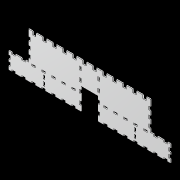
# Autodesk Inventor part: AluminumTopPlate
Saved by Autodesk Inventor 2021 (Build 250183000, 183)
## iProperties
Created: 2021-03-05
Part Number: AluminumTopPlate
Material: Aluminum 6061
Document SubType Name: Modeling
Designer: M3rob
Density: 2.7 g/cm^3
Appearance: Aluminum - Flat
Mass: 6715.1 g
Surface Area: 6765.43 cm^2
Volume: 2487.07 cm^3
Author: M3rob
Autodesk Inventor part; units mm, degrees
ref_plane "YZ Plane" through (0, 0, 0) normal (1, 0, 0) x (0, 1, 0)
ref_plane "XZ Plane" through (0, 0, 0) normal (0, 1, 0) x (-1, 0, 0)
ref_plane "XY Plane" through (0, 0, 0) normal (0, 0, 1) x (1, 0, 0)
sketch "Sketch1" plane through (0, 0, 0) normal (0, 0, 1) x (1, 0, 0)
  line L0 (-527.05, -334.01) -> (-527.05, 34.29) projected
  line L1 (-654.05, 34.29) -> (-654.05, -334.01) projected
  line L2 (-1206.5, -6.35) -> (-654.05, -6.35)
  line L3 (-1206.5, -6.35) -> (-1206.5, 120.65)
  line L4 (-1206.5, 120.65) -> (-1054.1, 120.65)
  line L5 (-1054.1, 120.65) -> (-1054.1, 339.09)
  line L6 (-1054.1, 339.09) -> (-127, 339.09)
  line L7 (-127, 339.09) -> (-127, 120.65)
  line L8 (-127, 120.65) -> (25.4, 120.65)
  line L9 (25.4, 120.65) -> (25.4, -6.35)
  line L10 (25.4, -6.35) -> (-527.05, -6.35)
  line L11 (-654.05, -6.35) -> (-654.05, 161.29)
  line L12 (-654.05, 161.29) -> (-527.05, 161.29)
  line L13 (-527.05, 161.29) -> (-527.05, -6.35)
  line L14 (-946.15, 339.09) -> (-920.75, 339.09) projected
  line L15 (-946.15, 339.09) -> (-946.15, 313.69) projected
  line L16 (-920.75, 313.69) -> (-946.15, 313.69) projected
  line L17 (-920.75, 339.09) -> (-920.75, 313.69) projected
  line L18 (-920.75, 339.09) -> (-869.95, 339.09) projected
  line L19 (-920.75, 339.09) -> (-920.75, 313.69) projected
  line L20 (-869.95, 313.69) -> (-920.75, 313.69) projected
  line L21 (-869.95, 339.09) -> (-869.95, 313.69) projected
  line L22 (-869.95, 339.09) -> (-844.55, 339.09) projected
  line L23 (-869.95, 339.09) -> (-869.95, 313.69) projected
  line L24 (-844.55, 313.69) -> (-869.95, 313.69) projected
  line L25 (-844.55, 339.09) -> (-844.55, 313.69) projected
  line L26 (-828.675, 339.09) -> (-828.675, 313.69) projected
  line L27 (-844.55, 339.09) -> (-825.8937, 339.09) projected
  line L28 (-844.55, 339.09) -> (-844.55, 313.69) projected
  line L29 (-825.8937, 313.69) -> (-844.55, 313.69) projected
  line L30 (-825.8937, 339.09) -> (-825.8937, 313.69) projected
  line L31 (-812.4063, 339.09) -> (-812.4063, 313.69) projected
  line L32 (-825.8937, 339.09) -> (-812.4063, 339.09) projected
  line L33 (-825.8937, 339.09) -> (-825.8937, 313.69) projected
  line L34 (-812.4063, 313.69) -> (-825.8937, 313.69) projected
  line L35 (-812.4063, 339.09) -> (-812.4063, 313.69) projected
  line L36 (-793.75, 339.09) -> (-793.75, 313.69) projected
  line L37 (-812.4063, 339.09) -> (-793.75, 339.09) projected
  line L38 (-812.4063, 339.09) -> (-812.4063, 313.69) projected
  line L39 (-793.75, 313.69) -> (-812.4063, 313.69) projected
  line L40 (-793.75, 339.09) -> (-793.75, 313.69) projected
  line L41 (-793.75, 339.09) -> (-768.35, 339.09) projected
  line L42 (-793.75, 339.09) -> (-793.75, 313.69) projected
  line L43 (-768.35, 313.69) -> (-793.75, 313.69) projected
  line L44 (-768.35, 339.09) -> (-768.35, 313.69) projected
  line L45 (-768.35, 339.09) -> (-717.55, 339.09) projected
  line L46 (-768.35, 339.09) -> (-768.35, 313.69) projected
  line L47 (-717.55, 313.69) -> (-768.35, 313.69) projected
  line L48 (-717.55, 339.09) -> (-717.55, 313.69) projected
  line L49 (-717.55, 339.09) -> (-692.15, 339.09) projected
  line L50 (-717.55, 339.09) -> (-717.55, 313.69) projected
  line L51 (-692.15, 313.69) -> (-717.55, 313.69) projected
  line L52 (-692.15, 339.09) -> (-692.15, 313.69) projected
  line L53 (-692.15, 339.09) -> (-641.35, 339.09) projected
  line L54 (-692.15, 339.09) -> (-692.15, 313.69) projected
  line L55 (-641.35, 313.69) -> (-692.15, 313.69) projected
  line L56 (-641.35, 339.09) -> (-641.35, 313.69) projected
  line L57 (-641.35, 339.09) -> (-615.95, 339.09) projected
  line L58 (-641.35, 339.09) -> (-641.35, 313.69) projected
  line L59 (-615.95, 313.69) -> (-641.35, 313.69) projected
  line L60 (-615.95, 339.09) -> (-615.95, 313.69) projected
  line L61 (-600.075, 339.09) -> (-600.075, 313.69) projected
  line L62 (-615.95, 339.09) -> (-597.2937, 339.09) projected
  line L63 (-615.95, 339.09) -> (-615.95, 313.69) projected
  line L64 (-597.2937, 313.69) -> (-615.95, 313.69) projected
  line L65 (-597.2937, 339.09) -> (-597.2937, 313.69) projected
  line L66 (-565.15, 339.09) -> (-539.75, 339.09) projected
  line L67 (-565.15, 339.09) -> (-565.15, 313.69) projected
  line L68 (-539.75, 313.69) -> (-565.15, 313.69) projected
  line L69 (-539.75, 339.09) -> (-539.75, 313.69) projected
  line L70 (-488.95, 339.09) -> (-463.55, 339.09) projected
  line L71 (-488.95, 339.09) -> (-488.95, 313.69) projected
  line L72 (-463.55, 313.69) -> (-488.95, 313.69) projected
  line L73 (-463.55, 339.09) -> (-463.55, 313.69) projected
  line L74 (-412.75, 339.09) -> (-387.35, 339.09) projected
  line L75 (-412.75, 339.09) -> (-412.75, 313.69) projected
  line L76 (-387.35, 313.69) -> (-412.75, 313.69) projected
  line L77 (-387.35, 339.09) -> (-387.35, 313.69) projected
  line L78 (-336.55, 339.09) -> (-311.15, 339.09) projected
  line L79 (-336.55, 339.09) -> (-336.55, 313.69) projected
  line L80 (-311.15, 313.69) -> (-336.55, 313.69) projected
  line L81 (-311.15, 339.09) -> (-311.15, 313.69) projected
  line L82 (-260.35, 339.09) -> (-234.95, 339.09) projected
  line L83 (-260.35, 339.09) -> (-260.35, 313.69) projected
  line L84 (-234.95, 313.69) -> (-260.35, 313.69) projected
  line L85 (-234.95, 339.09) -> (-234.95, 313.69) projected
  line L86 (-184.15, 339.09) -> (-158.75, 339.09) projected
  line L87 (-184.15, 339.09) -> (-184.15, 313.69) projected
  line L88 (-158.75, 313.69) -> (-184.15, 313.69) projected
  line L89 (-158.75, 339.09) -> (-158.75, 313.69) projected
  line L90 (-238.125, 92.075) -> (-250.825, 92.075) projected
  line L91 (-250.825, 66.675) -> (-250.825, 92.075) projected
  line L92 (-238.125, 66.675) -> (-250.825, 66.675) projected
  line L93 (-238.125, 92.075) -> (-238.125, 66.675) projected
  line L94 (-238.125, 47.625) -> (-250.825, 47.625) projected
  line L95 (-250.825, 22.225) -> (-250.825, 47.625) projected
  line L96 (-238.125, 22.225) -> (-250.825, 22.225) projected
  line L97 (-238.125, 47.625) -> (-238.125, 22.225) projected
  line L98 (-304.8, 107.95) -> (-304.8, 120.65) projected
  line L99 (-330.2, 120.65) -> (-304.8, 120.65) projected
  line L100 (-330.2, 107.95) -> (-330.2, 120.65) projected
  line L101 (-304.8, 107.95) -> (-330.2, 107.95) projected
  line L102 (-381, 107.95) -> (-381, 120.65) projected
  line L103 (-406.4, 120.65) -> (-381, 120.65) projected
  line L104 (-406.4, 107.95) -> (-406.4, 120.65) projected
  line L105 (-381, 107.95) -> (-406.4, 107.95) projected
  line L106 (-76.2, 107.95) -> (-76.2, 120.65) projected
  line L107 (-101.6, 120.65) -> (-76.2, 120.65) projected
  line L108 (-101.6, 107.95) -> (-101.6, 120.65) projected
  line L109 (-76.2, 107.95) -> (-101.6, 107.95) projected
  line L110 (0, 107.95) -> (0, 120.65) projected
  line L111 (-25.4, 120.65) -> (0, 120.65) projected
  line L112 (-25.4, 107.95) -> (-25.4, 120.65) projected
  line L113 (0, 107.95) -> (-25.4, 107.95) projected
  line L114 (25.4, 92.075) -> (12.7, 92.075) projected
  line L115 (12.7, 66.675) -> (12.7, 92.075) projected
  line L116 (25.4, 66.675) -> (12.7, 66.675) projected
  line L117 (25.4, 92.075) -> (25.4, 66.675) projected
  line L118 (0, -6.35) -> (0, 6.35) projected
  line L119 (-25.4, 6.35) -> (0, 6.35) projected
  line L120 (-25.4, -6.35) -> (-25.4, 6.35) projected
  line L121 (0, -6.35) -> (-25.4, -6.35) projected
  line L122 (-76.2, -6.35) -> (-76.2, 6.35) projected
  line L123 (-101.6, 6.35) -> (-76.2, 6.35) projected
  line L124 (-101.6, -6.35) -> (-101.6, 6.35) projected
  line L125 (-76.2, -6.35) -> (-101.6, -6.35) projected
  line L126 (-152.4, -6.35) -> (-152.4, 6.35) projected
  line L127 (-177.8, 6.35) -> (-152.4, 6.35) projected
  line L128 (-177.8, -6.35) -> (-177.8, 6.35) projected
  line L129 (-152.4, -6.35) -> (-177.8, -6.35) projected
  line L130 (-228.6, -6.35) -> (-228.6, 6.35) projected
  line L131 (-254, 6.35) -> (-228.6, 6.35) projected
  line L132 (-254, -6.35) -> (-254, 6.35) projected
  line L133 (-228.6, -6.35) -> (-254, -6.35) projected
  line L134 (-304.8, -6.35) -> (-304.8, 6.35) projected
  line L135 (-330.2, 6.35) -> (-304.8, 6.35) projected
  line L136 (-330.2, -6.35) -> (-330.2, 6.35) projected
  line L137 (-304.8, -6.35) -> (-330.2, -6.35) projected
  line L138 (-381, -6.35) -> (-381, 6.35) projected
  line L139 (-406.4, 6.35) -> (-381, 6.35) projected
  line L140 (-406.4, -6.35) -> (-406.4, 6.35) projected
  line L141 (-381, -6.35) -> (-406.4, -6.35) projected
  line L142 (-457.2, -6.35) -> (-457.2, 6.35) projected
  line L143 (-482.6, 6.35) -> (-457.2, 6.35) projected
  line L144 (-482.6, -6.35) -> (-482.6, 6.35) projected
  line L145 (-457.2, -6.35) -> (-482.6, -6.35) projected
  line L146 (-514.35, 59.69) -> (-527.05, 59.69) projected
  line L147 (-527.05, 34.29) -> (-527.05, 59.69) projected
  line L148 (-514.35, 34.29) -> (-527.05, 34.29) projected
  line L149 (-514.35, 59.69) -> (-514.35, 34.29) projected
  line L150 (-514.35, 135.89) -> (-527.05, 135.89) projected
  line L151 (-527.05, 110.49) -> (-527.05, 135.89) projected
  line L152 (-514.35, 110.49) -> (-527.05, 110.49) projected
  line L153 (-514.35, 135.89) -> (-514.35, 110.49) projected
  line L154 (-514.35, 212.09) -> (-527.05, 212.09) projected
  line L155 (-527.05, 186.69) -> (-527.05, 212.09) projected
  line L156 (-514.35, 186.69) -> (-527.05, 186.69) projected
  line L157 (-514.35, 212.09) -> (-514.35, 186.69) projected
  line L158 (-514.35, 288.29) -> (-527.05, 288.29) projected
  line L159 (-527.05, 262.89) -> (-527.05, 288.29) projected
  line L160 (-514.35, 262.89) -> (-527.05, 262.89) projected
  line L161 (-514.35, 288.29) -> (-514.35, 262.89) projected
  line L162 (-654.05, 288.29) -> (-666.75, 288.29) projected
  line L163 (-666.75, 262.89) -> (-666.75, 288.29) projected
  line L164 (-654.05, 262.89) -> (-666.75, 262.89) projected
  line L165 (-654.05, 288.29) -> (-654.05, 262.89) projected
  line L166 (-654.05, 212.09) -> (-666.75, 212.09) projected
  line L167 (-666.75, 186.69) -> (-666.75, 212.09) projected
  line L168 (-654.05, 186.69) -> (-666.75, 186.69) projected
  line L169 (-654.05, 212.09) -> (-654.05, 186.69) projected
  line L170 (-654.05, 135.89) -> (-666.75, 135.89) projected
  line L171 (-666.75, 110.49) -> (-666.75, 135.89) projected
  line L172 (-654.05, 110.49) -> (-666.75, 110.49) projected
  line L173 (-654.05, 135.89) -> (-654.05, 110.49) projected
  line L174 (-723.9, 120.65) -> (-723.9, 107.95) projected
  line L175 (-698.5, 107.95) -> (-723.9, 107.95) projected
  line L176 (-698.5, 120.65) -> (-698.5, 107.95) projected
  line L177 (-723.9, 120.65) -> (-698.5, 120.65) projected
  line L178 (-800.1, 120.65) -> (-800.1, 107.95) projected
  line L179 (-774.7, 107.95) -> (-800.1, 107.95) projected
  line L180 (-774.7, 120.65) -> (-774.7, 107.95) projected
  line L181 (-800.1, 120.65) -> (-774.7, 120.65) projected
  line L182 (-654.05, 59.69) -> (-666.75, 59.69) projected
  line L183 (-666.75, 34.29) -> (-666.75, 59.69) projected
  line L184 (-654.05, 34.29) -> (-666.75, 34.29) projected
  line L185 (-654.05, 59.69) -> (-654.05, 34.29) projected
  line L186 (-698.5, -6.35) -> (-698.5, 6.35) projected
  line L187 (-723.9, 6.35) -> (-698.5, 6.35) projected
  line L188 (-723.9, -6.35) -> (-723.9, 6.35) projected
  line L189 (-698.5, -6.35) -> (-723.9, -6.35) projected
  line L190 (-774.7, -6.35) -> (-774.7, 6.35) projected
  line L191 (-800.1, 6.35) -> (-774.7, 6.35) projected
  line L192 (-800.1, -6.35) -> (-800.1, 6.35) projected
  line L193 (-774.7, -6.35) -> (-800.1, -6.35) projected
  line L194 (-850.9, -6.35) -> (-850.9, 6.35) projected
  line L195 (-876.3, 6.35) -> (-850.9, 6.35) projected
  line L196 (-876.3, -6.35) -> (-876.3, 6.35) projected
  line L197 (-850.9, -6.35) -> (-876.3, -6.35) projected
  line L198 (-927.1, -6.35) -> (-927.1, 6.35) projected
  line L199 (-952.5, 6.35) -> (-927.1, 6.35) projected
  line L200 (-952.5, -6.35) -> (-952.5, 6.35) projected
  line L201 (-927.1, -6.35) -> (-952.5, -6.35) projected
  line L202 (-930.275, 47.625) -> (-942.975, 47.625) projected
  line L203 (-942.975, 22.225) -> (-942.975, 47.625) projected
  line L204 (-930.275, 22.225) -> (-942.975, 22.225) projected
  line L205 (-930.275, 47.625) -> (-930.275, 22.225) projected
  line L206 (-930.275, 92.075) -> (-942.975, 92.075) projected
  line L207 (-942.975, 66.675) -> (-942.975, 92.075) projected
  line L208 (-930.275, 66.675) -> (-942.975, 66.675) projected
  line L209 (-930.275, 92.075) -> (-930.275, 66.675) projected
  line L210 (-942.975, 92.075) -> (-942.975, 66.675) projected
  line L211 (-876.3, 120.65) -> (-876.3, 107.95) projected
  line L212 (-850.9, 107.95) -> (-876.3, 107.95) projected
  line L213 (-850.9, 120.65) -> (-850.9, 107.95) projected
  line L214 (-876.3, 120.65) -> (-850.9, 120.65) projected
  line L215 (-952.5, 120.65) -> (-952.5, 107.95) projected
  line L216 (-927.1, 107.95) -> (-952.5, 107.95) projected
  line L217 (-927.1, 120.65) -> (-927.1, 107.95) projected
  line L218 (-952.5, 120.65) -> (-927.1, 120.65) projected
  line L219 (-1028.7, 120.65) -> (-1028.7, 107.95) projected
  line L220 (-1003.3, 107.95) -> (-1028.7, 107.95) projected
  line L221 (-1003.3, 120.65) -> (-1003.3, 107.95) projected
  line L222 (-1028.7, 120.65) -> (-1003.3, 120.65) projected
  line L223 (-1003.3, -6.35) -> (-1003.3, 6.35) projected
  line L224 (-1028.7, 6.35) -> (-1003.3, 6.35) projected
  line L225 (-1028.7, -6.35) -> (-1028.7, 6.35) projected
  line L226 (-1003.3, -6.35) -> (-1028.7, -6.35) projected
  line L227 (-1079.5, -6.35) -> (-1079.5, 6.35) projected
  line L228 (-1104.9, 6.35) -> (-1079.5, 6.35) projected
  line L229 (-1104.9, -6.35) -> (-1104.9, 6.35) projected
  line L230 (-1079.5, -6.35) -> (-1104.9, -6.35) projected
  line L231 (-1155.7, -6.35) -> (-1155.7, 6.35) projected
  line L232 (-1181.1, 6.35) -> (-1155.7, 6.35) projected
  line L233 (-1181.1, -6.35) -> (-1181.1, 6.35) projected
  line L234 (-1155.7, -6.35) -> (-1181.1, -6.35) projected
  line L235 (-1193.8, 47.625) -> (-1206.5, 47.625) projected
  line L236 (-1206.5, 22.225) -> (-1206.5, 47.625) projected
  line L237 (-1193.8, 22.225) -> (-1206.5, 22.225) projected
  line L238 (-1193.8, 47.625) -> (-1193.8, 22.225) projected
  line L239 (-1193.8, 92.075) -> (-1206.5, 92.075) projected
  line L240 (-1206.5, 66.675) -> (-1206.5, 92.075) projected
  line L241 (-1193.8, 66.675) -> (-1206.5, 66.675) projected
  line L242 (-1193.8, 92.075) -> (-1193.8, 66.675) projected
  line L243 (-1181.1, 120.65) -> (-1181.1, 107.95) projected
  line L244 (-1155.7, 107.95) -> (-1181.1, 107.95) projected
  line L245 (-1155.7, 120.65) -> (-1155.7, 107.95) projected
  line L246 (-1181.1, 120.65) -> (-1155.7, 120.65) projected
  line L247 (-1104.9, 120.65) -> (-1104.9, 107.95) projected
  line L248 (-1079.5, 107.95) -> (-1104.9, 107.95) projected
  line L249 (-1079.5, 120.65) -> (-1079.5, 107.95) projected
  line L250 (-1104.9, 120.65) -> (-1079.5, 120.65) projected
  line L251 (-1041.4, 171.45) -> (-1054.1, 171.45) projected
  line L252 (-1054.1, 146.05) -> (-1054.1, 171.45) projected
  line L253 (-1041.4, 146.05) -> (-1054.1, 146.05) projected
  line L254 (-1041.4, 171.45) -> (-1041.4, 146.05) projected
  line L255 (-1041.4, 229.87) -> (-1054.1, 229.87) projected
  line L256 (-1054.1, 204.47) -> (-1054.1, 229.87) projected
  line L257 (-1041.4, 204.47) -> (-1054.1, 204.47) projected
  line L258 (-1041.4, 229.87) -> (-1041.4, 204.47) projected
  line L259 (-1041.4, 288.29) -> (-1054.1, 288.29) projected
  line L260 (-1054.1, 262.89) -> (-1054.1, 288.29) projected
  line L261 (-1041.4, 262.89) -> (-1054.1, 262.89) projected
  line L262 (-1041.4, 288.29) -> (-1041.4, 262.89) projected
  line L263 (-1104.9, 107.95) -> (-1079.5, 107.95) projected
  line L264 (-1022.35, 339.09) -> (-996.95, 339.09) projected
  line L265 (-1022.35, 339.09) -> (-1022.35, 313.69) projected
  line L266 (-996.95, 313.69) -> (-1022.35, 313.69) projected
  line L267 (-996.95, 339.09) -> (-996.95, 313.69) projected
  line L268 (25.4, 47.625) -> (12.7, 47.625) projected
  line L269 (12.7, 22.225) -> (12.7, 47.625) projected
  line L270 (25.4, 22.225) -> (12.7, 22.225) projected
  line L271 (25.4, 47.625) -> (25.4, 22.225) projected
  line L272 (-228.6, 107.95) -> (-228.6, 120.65) projected
  line L273 (-254, 120.65) -> (-228.6, 120.65) projected
  line L274 (-254, 107.95) -> (-254, 120.65) projected
  line L275 (-228.6, 107.95) -> (-254, 107.95) projected
  line L276 (-152.4, 107.95) -> (-152.4, 120.65) projected
  line L277 (-177.8, 120.65) -> (-152.4, 120.65) projected
  line L278 (-177.8, 107.95) -> (-177.8, 120.65) projected
  line L279 (-152.4, 107.95) -> (-177.8, 107.95) projected
  line L280 (-127, 171.45) -> (-139.7, 171.45) projected
  line L281 (-139.7, 146.05) -> (-139.7, 171.45) projected
  line L282 (-127, 146.05) -> (-139.7, 146.05) projected
  line L283 (-127, 171.45) -> (-127, 146.05) projected
  line L284 (-127, 229.87) -> (-139.7, 229.87) projected
  line L285 (-139.7, 204.47) -> (-139.7, 229.87) projected
  line L286 (-127, 204.47) -> (-139.7, 204.47) projected
  line L287 (-127, 229.87) -> (-127, 204.47) projected
  line L288 (-127, 288.29) -> (-139.7, 288.29) projected
  line L289 (-139.7, 262.89) -> (-139.7, 288.29) projected
  line L290 (-127, 262.89) -> (-139.7, 262.89) projected
  line L291 (-127, 288.29) -> (-127, 262.89) projected
  line L292 (-457.2, 107.95) -> (-457.2, 120.65) projected
  line L293 (-482.6, 120.65) -> (-457.2, 120.65) projected
  line L294 (-482.6, 107.95) -> (-482.6, 120.65) projected
  line L295 (-457.2, 107.95) -> (-482.6, 107.95) projected
  point P0 (0, 0)
  point P1 (-666.75, -6.35)
  point P2 (-514.35, -6.35)
  point P3 (-1123.5563, 120.65)
  point P4 (-517.6811, -6.35)
  point P5 (-663.4189, -6.35)
  dimension "d0" = 177.8
  constraints: 18 end point, 6 perpendicular, 5 vertical, 2 point on line, 21 other
extrude "Extrusion1" add sketch "Sketch1" along normal blind 7.9375 contours L0 L148 L149 L146 L13 L152 L153 L150 L12 L11 L170 L171 L172 L182 L183 L184 L1 L2 L186 L187 L188 L190 L191 L192 L194 L195 L196 L198 L199 L200 L223 L224 L225 L227 L228 L229 L231 L232 L233 L3 L237 L238 L235 L241 L242 L239 L4 L243 L244 L245 L247 L248 L249 L5 L253 L254 L251 L257 L258 L255 L261 L262 L259 L6 L265 L266 L267 L15 L16 L20 L24 L29 L34 L39 L43 L47 L51 L55 L59 L64 L65 L67 L68 L69 L71 L72 L73 L75 L76 L77 L79 L80 L81 L83 L84 L85 L87 L88 L89 L7 L288 L289 L290 L284 L285 L286 L280 L281 L282 L8 L108 L109 L106 L112 L113 L110 L9 L114 L115 L116 L268 L269 L270 L10 L118 L119 L120 L122 L123 L124 L126 L127 L128 L130 L131 L132 L134 L135 L136 L138 L139 L140 L142 L143 L144 | L65 L64 L61 L6 | L61 L64 L60 L6 | L6 L21 L20 L17 | L56 L55 L52 L6 | L6 L26 L29 L25 | L6 L30 L29 L26 | L48 L47 L44 L6 | L6 L31 L34 L30 | L6 L36 L39 L31
body "Solid1"
